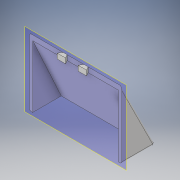
# Autodesk Inventor part: foot_cover_2_top
Saved by Autodesk Inventor 2018 (Build 220112000, 112)
## iProperties
Created: 2018-12-11
Part Number: foot_cover_2_top
Material: Generic
Document SubType Name: Modeling
Designer: jaspe
Density: 1 g/cm^3
Appearance: Default
Author: jaspe
Autodesk Inventor part; units mm, degrees
ref_plane "YZ Plane" through (0, 0, 0) normal (1, 0, 0) x (0, 1, 0)
ref_plane "XY Plane" through (0, 0, 0) normal (0, 0, 1) x (1, 0, 0)
sketch "Sketch1" plane through (0, 0, 0) normal (1, 0, 0) x (0, 1, 0)
  line L0 (0, 0) -> (0, -80)
  line L1 (0, 0) -> (80, 0) construction
  line L2 (0, -80) -> (40, -80)
  line L3 (0, -80) -> (40, -80) construction
  line L4 (40, -80) -> (0, 0)
  dimension "d0" = 80
  dimension "d1" = 90
  dimension "d2" = 40
  dimension "d3" = 0
  constraints: 10 end point, 3 horizontal, 2 equal length, 1 vertical
  measures "d0" distance of L0.start L0.end
  measures "d1" angle of L0 L1
  measures "d2" distance of L0.end L2.end
  measures "d3" distance between parallel lines of L2 L3
extrude "Extrusion1" add sketch "Sketch1" along normal blind 110
ref_plane "Work Plane1" through (106, 0, 0) normal (1, 0, 0) x (0, 0, -1)
sketch "Sketch2" plane through (106, 0, 0) normal (1, 0, 0) x (0, 0, -1)
  line L0 (0, 0) -> (80, 0) projected
  line L1 (80, 0) -> (80, 40) projected
  line L2 (80, 40) -> (0, 0) projected
  line L3 (0, 0) -> (80, 0) projected
  line L4 (80, 0) -> (80, 34)
  line L5 (80, 0) -> (80, 40) projected
  line L6 (80, 0) -> (114, 0) construction
  line L7 (80, 0) -> (6, 0)
  line L8 (80, 0) -> (154, 0) construction
  line L9 (6, 0) -> (80, 34)
  dimension "d7" = 34
  dimension "d8" = 90
  dimension "d9" = 74
  dimension "d10" = 180
  constraints: 10 end point, 2 collinear, 2 equal length, 2 horizontal
  measures "d7" distance of L0.end L4.end
  measures "d8" angle of L6 L4
  measures "d9" distance of L0.end L7.end
  measures "d10" angle of L7 L8
extrude "Extrusion2" cut sketch "Sketch2" against normal blind 102 contours L9 L1 L0
sketch "Sketch3" plane through (0, 0, -80) normal (0, -1, 0) x (1, 0, 0)
  line L0 (0, 80) -> (0, 0) construction
  line L1 (0, 80) -> (37.5, 80) construction
  line L2 (0, 80) -> (37.5, 80) construction
  line L3 (106, 74) -> (106, 0) construction
  line L4 (106, 0) -> (110, 0) construction
  line L5 (110, 80) -> (110, 0) construction
  line L6 (0, 80) -> (110, 80) construction
  line L7 (0, 80) -> (0, 0) construction
  line L8 (0, 0) -> (4, 0) construction
  line L9 (4, 0) -> (4, 74) construction
  line L10 (4, 74) -> (106, 74) construction
  line L11 (110, 80) -> (110, 0) construction
  line L12 (110, 80) -> (72.5, 80) construction
  line L13 (0, 80) -> (110, 80) construction
  line L14 (110, 80) -> (147.5, 80) construction
  line L15 (37.5, 80) -> (47.5, 80)
  line L16 (47.5, 80) -> (47.5, 74)
  line L17 (47.5, 74) -> (37.5, 74)
  line L18 (37.5, 74) -> (37.5, 80)
  line L19 (72.5, 80) -> (62.5, 80)
  line L20 (62.5, 80) -> (62.5, 74)
  line L21 (62.5, 74) -> (72.5, 74)
  line L22 (72.5, 74) -> (72.5, 80)
  dimension "d13" = 37.5
  dimension "d14" = 0
  dimension "d17" = 37.5
  dimension "d18" = 180
  dimension "d21" = 10
  dimension "d22" = 6
  dimension "d23" = 10
  dimension "d24" = 6
  constraints: 24 end point, 5 horizontal, 4 parallel, 3 collinear, 2 perpendicular
  measures "d13" distance of L0.start L1.end
  measures "d14" distance between parallel lines of L1 L2
  measures "d17" distance of L5.start L12.end
  measures "d18" angle of L12 L14
  measures "d21" distance of L16.end L17.end
  measures "d22" distance of L15.end L16.end
  measures "d23" distance of L21.end L20.end
  measures "d24" distance of L20.end L19.end
extrude "Extrusion3" add sketch "Sketch3" along normal blind 4.33
draft "FaceDraft1" angle 30 pull direction (0, 1, 0) faces at (47.5, -1.4433, -2) fixed edges at (47.5, -4.33, -3)
draft "FaceDraft2" angle 30 pull direction (0, 1, 0) faces at (37.5, -1.4433, -4) fixed edges at (37.5, -4.33, -3)
draft "FaceDraft4" angle -30 pull direction (0, -1, 0) faces at (72.5, -1.4433, -4) fixed edges at (72.5, -4.33, -3)
fillet "Fillet2" radius 2 5 edges at (110, 20, -40) (110, 20, -80) (55, 40, -80) (0, 20, -80) (0, 20, -40)
draft "FaceDraft5" angle 30 pull direction (0, 1, 0) faces at (62.5, -1.4433, -2) fixed edges at (62.5, -4.33, -3)
body "Solid1"
